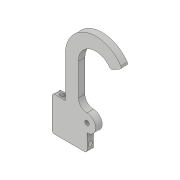
# Autodesk Inventor part: CLB_041_ScissorHook
Saved by Autodesk Inventor 2018 (Build 220112000, 112)
## iProperties
Created: 2020-02-08
Part Number: CLB_041_ScissorHook
Material: Generic
Document SubType Name: Modeling
Designer: Cooper
Density: 1 g/cm^3
Appearance: Default
Mass: 52.8359 g
Surface Area: 173.603 cm^2
Volume: 52.8359 cm^3
Author: Cooper
Autodesk Inventor part; units mm, degrees
ref_plane "YZ Plane" through (0, 0, 0) normal (1, 0, 0) x (0, 1, 0)
ref_plane "XZ Plane" through (0, 0, 0) normal (0, 1, 0) x (-1, 0, 0)
ref_plane "XY Plane" through (0, 0, 0) normal (0, 0, 1) x (1, 0, 0)
sketch "Sketch1" plane through (0, 0, 0) normal (0, 0, 1) x (1, 0, 0)
  line L0 (0, 0) -> (50.8, 0)
  line L1 (0, 0) -> (0, 50.8)
  line L2 (0, 50.8) -> (19.05, 50.8)
  arc A0 (101.9948, 132.2372) -> (19.05, 110.0122) centre (63.5, 110.0122) ccw
  arc A1 (85.497, 122.7122) -> (38.1, 110.0122) centre (63.5, 110.0122) ccw
  line L3 (85.497, 122.7122) -> (101.9948, 132.2372)
  line L4 (19.05, 110.0122) -> (19.05, 50.8)
  line L5 (38.1, 110.0122) -> (38.1, 63.5)
  arc A2 (50.8, 25.4) -> (50.8, 50.8) centre (50.8, 38.1) ccw
  arc A3 (38.1, 63.5) -> (50.8, 50.8) centre (50.8, 63.5) ccw
  line L6 (50.8, 0) -> (50.8, 25.4)
  dimension "d5" = 25.4
  dimension "d6" = 44.45
  dimension "d38" = 50.8
  dimension "d65" = 30
  dimension "d84" = 12.7
  dimension "d85" = 12.7
  dimension "d89" = 73.025
  dimension "d90" = 19.05
  dimension "d99" = 0
  dimension "d123" = 50.8
  dimension "d124" = 25.4
  constraints: 14 end point, 8 point on circle, 4 centre point, 4 tangent, 4 vertical, 2 horizontal, 2 line through centre, 1 coincident
  measures "d5" radius of A1
  measures "d6" radius of A0
  measures "d38" distance between parallel lines of L0 L2
  measures "d65" angle of L3 L2
  measures "d84" radius of A2
  measures "d85" radius of A3
  measures "d89" distance of A2.centre A0.centre
  measures "d90" distance of L1.end L2.end
  measures "d99" horizontal distance of A2.centre A3.centre
  measures "d123" distance of L0.start L0.end
  measures "d124" distance of L0.end L6.end
extrude "Extrusion1" add sketch "Sketch1" along normal blind 9.525
sketch "Sketch11" plane through (0, 0, 9.525) normal (0, 0, 1) x (1, 0, 0)
  line L0 (0, 0) -> (50.8, 0) projected
  arc A0 (50.8, 25.4) -> (50.8, 50.8) centre (50.8, 38.1) ccw projected
  arc A1 (38.1, 63.5) -> (50.8, 50.8) centre (50.8, 63.5) ccw projected
  line L1 (38.1, 63.5) -> (38.1, 110.0122) projected
  arc A2 (85.497, 122.7122) -> (38.1, 110.0122) centre (63.5, 110.0122) ccw projected
  line L2 (85.497, 122.7122) -> (101.9948, 132.2372) projected
  arc A3 (101.9948, 132.2372) -> (19.05, 110.0122) centre (63.5, 110.0122) ccw projected
  line L3 (19.05, 110.0122) -> (19.05, 50.8) projected
  line L4 (19.05, 50.8) -> (0, 50.8) projected
  line L5 (0, 50.8) -> (0, 0) projected
  line L6 (50.8, 0) -> (50.8, 25.4) projected
  constraints: 1 coincident
hole "Hole3" at (50.8, 38.1, 9.525) direction (0, 0, -1) diameter 6.35 end through all
sketch "Sketch12" plane through (0, 50.8, 0) normal (0, 1, 0) x (1, 0, 0)
  line L0 (19.05, 0) -> (0, 0) projected
  line L1 (0, 0) -> (0, -9.525) projected
  line L2 (19.05, -9.525) -> (0, -9.525) projected
  line L3 (19.05, 0) -> (19.05, -9.525) projected
  point P0 (9.525, -4.7625)
  dimension "d108" = 4.7625
  dimension "d109" = 4.7625
  dimension "d110" = 9.525
  measures "d108" distance from line of L0 point (9.525, -4.763)
  measures "d109" distance from line of L2 point (9.525, -4.763)
  measures "d110" distance from line of point (9.525, -4.763) L1
sketch "Sketch14" plane through (50.8, 0, 0) normal (1, 0, 0) x (0, 0, -1)
  line L0 (0, 0) -> (0, 25.4) projected
  line L1 (0, 25.4) -> (-9.525, 25.4) projected
  line L2 (-9.525, 0) -> (-9.525, 25.4) projected
  line L3 (0, 0) -> (-9.525, 0) projected
  point P0 (-4.7625, 9.525)
  dimension "d125" = 4.7625
  dimension "d126" = 4.7625
  dimension "d127" = 9.525
  measures "d125" distance from line of L2 point (-4.763, 9.525)
  measures "d126" distance from line of L0 point (-4.763, 9.525)
  measures "d127" distance from line of L3 point (-4.763, 9.525)
hole "Hole5" at (50.8, 9.525, 4.7625) direction (-0.7071, 0.7071, 0) diameter 5.5626 end through all both
fillet "Fillet7" radius 3.175 5 edges at (50.8, 0, 4.7625) (0, 0, 4.7625) (0, 50.8, 4.7625) (85.497, 122.7122, 4.7625) (101.9948, 132.2372, 4.7625)
sketch "Sketch15" plane through (0, 0, 9.525) normal (0, 0, 1) x (1, 0, 0)
  arc A0 (99.1393, 130.5885) -> (100.1712, 135.1325) centre (97.5518, 133.3382) ccw projected
  arc A1 (100.1712, 135.1325) -> (19.05, 110.0122) centre (63.5, 110.0122) ccw projected
  line L0 (19.05, 110.0122) -> (19.05, 50.8) projected
  line L1 (19.05, 50.8) -> (3.175, 50.8) projected
  arc A2 (3.175, 50.8) -> (0, 47.625) centre (3.175, 47.625) ccw projected
  line L2 (0, 47.625) -> (0, 3.175) projected
  arc A3 (0, 3.175) -> (3.175, 0) centre (3.175, 3.175) ccw projected
  line L3 (3.175, 0) -> (47.625, 0) projected
  arc A4 (47.625, 0) -> (50.8, 3.175) centre (47.625, 3.175) ccw projected
  line L4 (50.8, 3.175) -> (50.8, 25.4) projected
  arc A5 (50.8, 25.4) -> (50.8, 50.8) centre (50.8, 38.1) ccw projected
  arc A6 (38.1, 63.5) -> (50.8, 50.8) centre (50.8, 63.5) ccw projected
  line L5 (38.1, 63.5) -> (38.1, 110.0122) projected
  arc A7 (83.9497, 125.0777) -> (38.1, 110.0122) centre (63.5, 110.0122) ccw projected
  arc A8 (83.9497, 125.0777) -> (88.0934, 124.2112) centre (86.5059, 126.9608) ccw projected
  line L6 (88.0934, 124.2112) -> (99.1393, 130.5885) projected
  circle A9 centre (50.8, 38.1) radius 3.175 projected
  line L7 (-3.175, 3.175) -> (-3.175, 47.625)
  arc A10 (3.175, 53.975) -> (-3.175, 47.625) centre (3.175, 47.625) ccw
  line L8 (3.175, 53.975) -> (15.875, 53.975)
  line L9 (15.875, 53.975) -> (15.875, 110.0122)
  arc A11 (102.7905, 136.9268) -> (15.875, 110.0122) centre (63.5, 110.0122) ccw
  arc A12 (100.7268, 127.8389) -> (102.7905, 136.9268) centre (97.5518, 133.3382) ccw
  line L10 (100.7268, 127.8389) -> (89.6809, 121.4616)
  arc A13 (81.3935, 123.1945) -> (89.6809, 121.4616) centre (86.5059, 126.9608) ccw
  arc A14 (81.3935, 123.1945) -> (41.275, 110.0122) centre (63.5, 110.0122) ccw
  line L11 (41.275, 110.0122) -> (41.275, 63.5)
  arc A15 (41.275, 63.5) -> (50.8, 53.975) centre (50.8, 63.5) ccw
  arc A16 (53.975, 22.5457) -> (50.8, 53.975) centre (50.8, 38.1) ccw
  line L12 (53.975, 22.5457) -> (53.975, 3.175)
  arc A17 (47.625, -3.175) -> (53.975, 3.175) centre (47.625, 3.175) ccw
  line L13 (47.625, -3.175) -> (3.175, -3.175)
  arc A18 (-3.175, 3.175) -> (3.175, -3.175) centre (3.175, 3.175) ccw
  point P0 (0, 0)
  dimension "d138" = 3.175
  constraints: 18 point on circle, 14 end point, 9 centre point, 15 other
  measures "d138" distance between parallel lines of L2 L7
body "Solid1"
